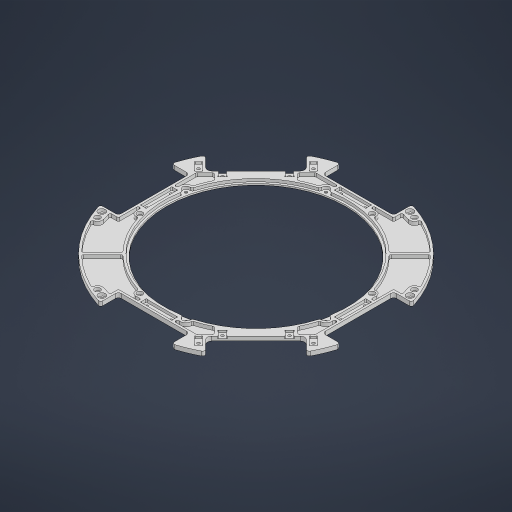
# Autodesk Inventor part: BasePlate
Saved by Autodesk Inventor 2024.2 (Build 282272000, 272)
## iProperties
Created: 2023-12-21
Part Number: BasePlate
Material: 一般
Document SubType Name: Modeling
Designer: Hanaoka
Density: 1 g/cm^3
Appearance: 既定
Author: Hanaoka
Autodesk Inventor part; units mm, degrees
(part 1 of 2)
ref_plane "YZ Plane" through (0, 0, 0) normal (1, 0, 0) x (0, 1, 0)
ref_plane "XZ Plane" through (0, 0, 0) normal (0, 1, 0) x (-1, 0, 0)
ref_plane "XY Plane" through (0, 0, 0) normal (0, 0, 1) x (1, 0, 0)
derived "MotorMount_main.ipt"
sketch "スケッチ4" plane through (-11, -15, 0) normal (0, -1, 0) x (1, 0, 0)
  circle A0 centre (19.5, 2) radius 0.8
  circle A1 centre (2.5, 2) radius 0.8
  line L0 (22, 0) -> (0, 0)
  line L1 (0, 0) -> (0, 4)
  line L2 (22, 4) -> (0, 4)
  line L3 (22, 0) -> (22, 4)
  circle A2 centre (11, -66) radius 90 construction
  line L4 (2.5, 2) -> (19.5, 2) construction
  line L5 (11, 2) -> (11, -66) construction
  circle A3 centre (11, -66) radius 88
  line L6 (-14, 18.374167) -> (-14, 7.5)
  line L7 (-12, 5.5) -> (34, 5.5)
  line L8 (36, 7.5) -> (36, 18.374167)
  arc A4 (-14, 7.5) -> (-12, 5.5) centre (-12, 7.5) ccw
  arc A5 (34, 5.5) -> (36, 7.5) centre (34, 7.5) ccw
  line L9 (0, 0) -> (22, 0)
  line L10 (22, 0) -> (22, 4)
  line L11 (22, 4) -> (0, 4)
  line L12 (0, 4) -> (0, 0)
  circle A6 centre (19.5, 2) radius 1
  circle A7 centre (2.5, 2) radius 1
  circle A8 centre (-57, -74.5) radius 1
  line L13 (-59, -77) -> (-55, -77)
  line L14 (-57, -74.5) -> (-57, -57.5) construction
  line L15 (-59, -55) -> (-59, -77)
  line L16 (-55, -55) -> (-59, -55)
  line L17 (-55, -77) -> (-55, -55)
  line L18 (-60.5, -89) -> (-60.5, -43)
  circle A9 centre (-57, -57.5) radius 1
  arc A10 (-62.5, -91) -> (-60.5, -89) centre (-62.5, -89) ccw
  line L19 (-62.5, -41) -> (-73.374167, -41)
  arc A11 (-60.5, -43) -> (-62.5, -41) centre (-62.5, -43) ccw
  line L20 (-73.374167, -91) -> (-62.5, -91)
  circle A12 centre (19.5, -134) radius 1
  line L21 (22, -136) -> (22, -132)
  line L22 (19.5, -134) -> (2.5, -134) construction
  line L23 (0, -136) -> (22, -136)
  line L24 (0, -132) -> (0, -136)
  line L25 (22, -132) -> (0, -132)
  line L26 (34, -137.5) -> (-12, -137.5)
  circle A13 centre (2.5, -134) radius 1
  arc A14 (36, -139.5) -> (34, -137.5) centre (34, -139.5) ccw
  line L27 (-14, -139.5) -> (-14, -150.374167)
  arc A15 (-12, -137.5) -> (-14, -139.5) centre (-12, -139.5) ccw
  line L28 (36, -150.374167) -> (36, -139.5)
  circle A16 centre (79, -57.5) radius 1
  line L29 (81, -55) -> (77, -55)
  line L30 (79, -57.5) -> (79, -74.5) construction
  line L31 (81, -77) -> (81, -55)
  line L32 (77, -77) -> (81, -77)
  line L33 (77, -55) -> (77, -77)
  line L34 (82.5, -43) -> (82.5, -89)
  circle A17 centre (79, -74.5) radius 1
  arc A18 (84.5, -41) -> (82.5, -43) centre (84.5, -43) ccw
  line L35 (84.5, -91) -> (95.374167, -91)
  arc A19 (82.5, -89) -> (84.5, -91) centre (84.5, -89) ccw
  line L36 (95.374167, -41) -> (84.5, -41)
  arc A20 (77.707107, -55) -> (77, -55.707107) centre (77.353553, -55.353553) ccw
  line L37 (77.353553, -55.353553) -> (77.353553, -55) construction
  line L38 (77.353553, -55.353553) -> (77, -55.353553) construction
  line L39 (77.353553, -55.353553) -> (77, -55) construction
  line L40 (80.646447, -55) -> (80.646447, -55.353553) construction
  line L41 (80.646447, -55.353553) -> (81, -55.353553) construction
  line L42 (77.353553, -77) -> (77.353553, -76.646447) construction
  line L43 (77.353553, -76.646447) -> (77, -76.646447) construction
  line L44 (81, -76.646447) -> (80.646447, -76.646447) construction
  line L45 (80.646447, -76.646447) -> (80.646447, -77) construction
  line L46 (81, -77) -> (80.646447, -76.646447) construction
  line L47 (77.353553, -76.646447) -> (77, -77) construction
  line L48 (81, -55) -> (80.646447, -55.353553) construction
  arc A21 (81, -55.707107) -> (80.292893, -55) centre (80.646447, -55.353553) ccw
  arc A22 (80.292893, -77) -> (81, -76.292893) centre (80.646447, -76.646447) ccw
  arc A23 (77, -76.292893) -> (77.707107, -77) centre (77.353553, -76.646447) ccw
  arc A24 (21.292893, 0) -> (22, 0.707107) centre (21.646447, 0.353553) ccw
  arc A25 (22, 3.292893) -> (21.292893, 4) centre (21.646447, 3.646447) ccw
  arc A26 (0, 0.707107) -> (0.707107, 0) centre (0.353553, 0.353553) ccw
  arc A27 (0.707107, 4) -> (0, 3.292893) centre (0.353553, 3.646447) ccw
  arc A28 (-55, -55.707107) -> (-55.707107, -55) centre (-55.353553, -55.353553) ccw
  arc A29 (-58.292893, -55) -> (-59, -55.707107) centre (-58.646447, -55.353553) ccw
  arc A30 (-55.707107, -77) -> (-55, -76.292893) centre (-55.353553, -76.646447) ccw
  arc A31 (-59, -76.292893) -> (-58.292893, -77) centre (-58.646447, -76.646447) ccw
  arc A32 (0.707107, -132) -> (0, -132.707107) centre (0.353553, -132.353553) ccw
  arc A33 (0, -135.292893) -> (0.707107, -136) centre (0.353553, -135.646447) ccw
  arc A34 (22, -132.707107) -> (21.292893, -132) centre (21.646447, -132.353553) ccw
  arc A35 (21.292893, -136) -> (22, -135.292893) centre (21.646447, -135.646447) ccw
  point P0 (11, 0)
  point P1 (-14, 5.5)
  point P2 (36, 5.5)
  point P3 (-57, -66)
  point P4 (-60.5, -91)
  point P5 (-60.5, -41)
  point P6 (11, -134)
  point P7 (36, -137.5)
  point P8 (-14, -137.5)
  point P9 (79, -66)
  point P10 (82.5, -41)
  point P11 (82.5, -91)
  point P12 (22, -135.292893)
  point P13 (21.292893, -136)
  point P14 (0.707107, -136)
  point P15 (0, -135.292893)
  point P16 (0, -132.707107)
  point P17 (0.707107, -132)
  point P18 (21.292893, -132)
  point P19 (22, -132.707107)
  point P20 (-58.292893, -77)
  point P21 (-59, -76.292893)
  point P22 (-59, -55.707107)
  point P23 (-58.292893, -55)
  point P24 (-55.707107, -55)
  point P25 (-55, -55.707107)
  point P26 (-55, -76.292893)
  point P27 (-55.707107, -77)
  point P28 (0, 3.292893)
  point P29 (0.707107, 4)
  point P30 (21.292893, 4)
  point P31 (22, 3.292893)
  point P32 (22, 0.707107)
  point P33 (21.292893, 0)
  point P34 (0.707107, 0)
  point P35 (0, 0.707107)
  dimension "d4" = 180
  dimension "d5" = 68
  dimension "d6" = 176
  dimension "d11" = 1.5
  dimension "d12" = 50
  dimension "d13" = 2
  dimension "d14" = 2
  dimension "d17" = 360
  dimension "d31" = 0.5
  dimension "d32" = 0.5
  dimension "d35" = 360
  constraints: 90 end point, 50 point on circle, 34 centre point, 32 point on line, 13 coincident, 8 equal length, 6 perpendicular, 5 equal radius, 4 horizontal, 4 tangent, 4 vertical, 3 parallel, 1 midpoint, 190 other
  measures "d4" diameter of A2
  measures "d5" distance of L5.start L5.end
  measures "d6" diameter of A3
  measures "d11" distance between parallel lines of L7 L2
  measures "d12" distance of point (-14, 5.5) point (36, 5.5)
  measures "d13" radius of A4
  measures "d14" diameter of A7
  measures "d31" radius of A20
  measures "d32" distance of L37.start L29.end
extrude "押し出し2" add sketch "スケッチ4" along normal blind 1 contours A24 L0 | L0 L1 L2 L3 | L3 A24 | A26 L0 | L3 A25 | A26 L1 | L2 A25 | A27 L1 | L2 A27 | L36 A18 L34 A19 L35 A3 L28 A14 L26 A15 L27 L20 A10 L18 A11 L19 L6 A4 L7 A5 L8 | A6 | A7 | L15 L16 L17 L13 | A31 L15 | L13 A31 | L13 A30 | A29 L15 | L17 A30 | A29 L16 | L17 A28 | A28 L16 | L23 L24 L25 L21 | A35 L23 | L21 A35 | L21 A34 | A33 L23 | L25 A34 | A33 L24 | L25 A32 | A32 L24 | L31 L32 L33 L29 | A21 L31 | L29 A21 | L29 A20 | A22 L31 | L33 A20 | A22 L32 | L33 A23 | A23 L32
extrude "押し出し3" add sketch "スケッチ4" against normal blind 2 contours L36 A18 L34 A19 L35 A3 L28 A14 L26 A15 L27 L20 A10 L18 A11 L19 L6 A4 L7 A5 L8
fillet "フィレット1" radius 1.5 8 edges at (-84.3742, -14.5, -41) (-25, -14.5, 18.3742) (25, -14.5, 18.3742) (84.3742, -14.5, -41) (84.3742, -14.5, -91) (25, -14.5, -150.3742) (-25, -14.5, -150.3742) (-84.3742, -14.5, -91)
sketch "溝切り" plane through (-23, -13, 5.5) normal (0, 1, 0) x (1, 0, 0)
  circle A0 centre (102.548727, 100) radius 2.5
  line L0 (96.5, 96.5) -> (105.340755, 96.5)
  arc A1 (106.76863, 98.459538) -> (49.959538, 155.26863) centre (23, 71.5) ccw
  circle A2 centre (102.548727, 100) radius 3.5 construction
  line L1 (85.225397, 133.725397) -> (-39.225397, 9.274603) construction
  arc A3 (-60.76863, 44.540462) -> (-3.959538, -12.26863) centre (23, 71.5) ccw
  circle A4 centre (51.5, 151.048727) radius 2.5
  circle A5 centre (51.5, 151.048727) radius 3.5 construction
  line L2 (-39.225397, 133.725397) -> (85.225397, 9.274603) construction
  arc A6 (49.959538, -12.26863) -> (106.76863, 44.540462) centre (23, 71.5) ccw
  arc A7 (-3.959538, 155.26863) -> (-60.76863, 98.459538) centre (23, 71.5) ccw
  circle A8 centre (-5.5, -8.048727) radius 2.5
  circle A9 centre (-5.5, -8.048727) radius 3.5 construction
  circle A10 centre (-56.548727, 43) radius 3.5 construction
  circle A11 centre (-56.548727, 43) radius 2.5
  circle A12 centre (102.548727, 100) radius 1.3
  circle A13 centre (51.5, 151.048727) radius 1.3
  circle A14 centre (-56.548727, 43) radius 1.3
  circle A15 centre (-5.5, -8.048727) radius 1.3
  circle A16 centre (23, 71.5) radius 63
  line L3 (-54.339215, 113.483876) -> (-46.914594, 106.059255)
  line L4 (-42.671953, 106.059255) -> (-11.559255, 137.171953)
  line L5 (-11.559255, 141.414594) -> (-18.983876, 148.839215)
  arc A17 (-46.914594, 106.059255) -> (-42.671953, 106.059255) centre (-44.793273, 108.180575) ccw
  arc A18 (-11.559255, 137.171953) -> (-11.559255, 141.414594) centre (-13.680575, 139.293273) ccw
  circle A19 centre (-41.964846, 136.464846) radius 21 construction
  line L6 (64.983876, -5.839215) -> (57.559255, 1.585406)
  line L7 (57.559255, 5.828047) -> (88.671953, 36.940745)
  line L8 (92.914594, 36.940745) -> (100.339215, 29.516124)
  arc A20 (57.559255, 5.828047) -> (57.559255, 1.585406) centre (59.680575, 3.706727) ccw
  arc A21 (92.914594, 36.940745) -> (88.671953, 36.940745) centre (90.793273, 34.819425) ccw
  circle A22 centre (8.265706, 135.321239) radius 2.5 construction
  circle A23 centre (8.265706, 135.321239) radius 1
  line L9 (8.265706, 135.321239) -> (23, 71.5) construction
  arc A24 (10.701631, 135.883617) -> (5.829781, 134.758862) centre (8.265706, 135.321239) ccw
  line L10 (5.829781, 134.758862) -> (6.403321, 132.274586)
  line L11 (10.701631, 135.883617) -> (11.275171, 133.399341)
  circle A25 centre (-40.821239, 86.234294) radius 2.5 construction
  circle A26 centre (-40.821239, 86.234294) radius 1
  arc A27 (-40.258862, 88.670219) -> (-41.383617, 83.798369) centre (-40.821239, 86.234294) ccw
  line L12 (-40.258862, 88.670219) -> (-37.774586, 88.096679)
  line L13 (-41.383617, 83.798369) -> (-38.899341, 83.224829)
  circle A28 centre (86.821239, 56.765706) radius 2.5 construction
  circle A29 centre (86.821239, 56.765706) radius 1
  arc A30 (86.258862, 54.329781) -> (87.383617, 59.201631) centre (86.821239, 56.765706) ccw
  line L14 (86.258862, 54.329781) -> (83.774586, 54.903321)
  line L15 (87.383617, 59.201631) -> (84.899341, 59.775171)
  line L16 (35.298369, 7.116383) -> (34.724829, 9.600659)
  line L17 (40.170219, 8.241138) -> (39.596679, 10.725414)
  circle A31 centre (37.734294, 7.678761) radius 2.5 construction
  circle A32 centre (37.734294, 7.678761) radius 1
  arc A33 (35.298369, 7.116383) -> (40.170219, 8.241138) centre (37.734294, 7.678761) ccw
  circle A34 centre (23, 71.5) radius 64.5
  line L18 (-48.5, 94.5) -> (-48.5, 96.330952) construction
  line L19 (-48.5, 96.330952) -> (-58.01901, 105.849963) construction
  line L20 (-48.5, 94.5) -> (-48.5, 48.5)
  line L21 (0, 143) -> (-1.830952, 143) construction
  line L22 (-1.830952, 143) -> (-11.349963, 152.51901) construction
  arc A35 (-60.76863, 98.459538) -> (-59.340755, 96.5) centre (-59.340755, 98) ccw
  line L23 (-59.340755, 96.5) -> (-50.5, 96.5)
  arc A36 (-48.5, 94.5) -> (-50.5, 96.5) centre (-50.5, 94.5) ccw
  arc A37 (-2, 153.840755) -> (-3.959538, 155.26863) centre (-3.5, 153.840755) ccw
  line L24 (-2, 145) -> (-2, 153.840755)
  arc A38 (-2, 145) -> (0, 143) centre (0, 145) ccw
  line L25 (46, 143) -> (0, 143)
  point P0 (23, 5.5)
  point P1 (-44.793273, 103.937934)
  point P2 (-9.437934, 139.293273)
  point P3 (100.339215, 29.516124)
  point P4 (39.596679, 10.725414)
  point P5 (34.724829, 9.600659)
  point P6 (84.899341, 59.775171)
  point P7 (83.774586, 54.903321)
  point P8 (-38.899341, 83.224829)
  point P9 (-37.774586, 88.096679)
  point P10 (-40.362021, 83.562515)
  point P11 (35.062515, 8.137979)
  point P12 (39.934365, 9.262734)
  point P13 (85.237266, 54.565635)
  point P14 (86.362021, 59.437485)
  point P15 (10.937485, 134.862021)
  point P16 (6.065635, 133.737266)
  point P17 (-39.237266, 88.434365)
  point P18 (-50.626904, 109.771565)
  point P19 (-11.349963, 152.51901)
  dimension "d20" = 5
  dimension "d22" = 7
  dimension "d23" = 2.6
  dimension "d28" = 126
  dimension "d37" = 50
  dimension "d38" = 3
  dimension "d39" = 42
  dimension "d40" = 13.5
  dimension "d45" = 2
  dimension "d46" = 5
  dimension "d47" = 32
  dimension "d48" = 1.5
  dimension "d102" = 8
  constraints: 42 end point, 38 symmetric about line, 31 centre point, 25 point on circle, 18 coincident, 11 tangent, 7 parallel, 5 equal radius, 5 point on line, 2 midpoint, 1 collinear, 1 vertical, 17 other
  measures "d20" diameter of A0
  measures "d22" diameter of A2
  measures "d23" diameter of A12
  measures "d28" diameter of A16
  measures "d37" distance of point (-44.793, 103.938) point (-9.438, 139.293)
  measures "d38" radius of A17
  measures "d39" diameter of A19
  measures "d40" distance from line of L5.end L4
  measures "d45" diameter of A23
  measures "d46" diameter of A22
  measures "d47" angle of L2 L9
  measures "d48" radial gap between concentric circles of A16 A34
  measures "d102" distance from line of point (-50.627, 109.772) L19
extrude "押し出し4" cut sketch "溝切り" against normal up to surface (3 mm away) contours A12 | A13 | A14 | A15
extrude "押し出し5" cut sketch "溝切り" against normal blind 2 contours A0 | A4 | A8 | A11 | A15 | A16 | A16 L11 A34 L15 | A16 L10 A34 L11 | L15 A34 L14 A16 | A16 L12 A34 L10 | A34 L10 A24 L11 | L14 A34 L17 A16 | L15 A30 L14 A34 | A16 L13 A34 L12 | L17 A34 L16 A16 | A16 L16 A34 L13 | A34 L13 A27 L12 | L17 A33 L16 A34
extrude "押し出し6" cut sketch "溝切り" against normal up to surface (3 mm away) contours L6 A20 L7 A21 L8 A6 | L5 A18 L4 A17 L3 A7 | A16 | A23 | A29 | A32 | A26
fillet "フィレット2" radius 1.5 4 edges at (-77.3392, -14.5, -107.9839) (-41.9839, -14.5, -143.3392) (41.9839, -14.5, 11.3392) (77.3392, -14.5, -24.0161)
fillet "フィレット3" radius 1.5 8 edges at (-62.2373, -14, -82.9344) (-63.362, -14, -78.0625) (-16.9344, -14, -128.2373) (-12.0625, -14, -129.362) (63.362, -14, -53.9375) (62.2373, -14, -49.0656) (12.0625, -14, -2.638) (16.9344, -14, -3.7627)
sketch "シャフト用はめ穴" plane through (-23, -13, -137.5) normal (0, 1, 0) x (1, 0, 0)
  circle A0 centre (-54.526174, -105.114614) radius 1
  circle A1 centre (-54.526174, -105.114614) radius 2
  circle A2 centre (-41.936507, -88) radius 2
  circle A3 centre (-41.936507, -88) radius 1
  circle A4 centre (-56.548727, -100) radius 2.5
  circle A5 centre (23, -71.5) radius 63
  arc A6 (-56.548727, -100) -> (-54.526174, -105.114614) centre (23, -71.5) ccw construction
  line L0 (85.225397, -9.274603) -> (-39.225397, -133.725397) construction
  line L1 (-39.225397, -9.274603) -> (85.225397, -133.725397) construction
  circle A7 centre (-10.614614, -149.026174) radius 1
  circle A8 centre (-10.614614, -149.026174) radius 2
  circle A9 centre (-41.936507, -88) radius 2.5 construction
  arc A10 (-40.607766, -60.808783) -> (33.691217, -135.107766) centre (23, -71.5) ccw
  line L2 (-43.707107, -82.5) -> (-46.292893, -82.5)
  circle A11 centre (6.5, -136.436507) radius 2
  circle A12 centre (6.5, -136.436507) radius 1
  circle A13 centre (6.5, -136.436507) radius 2.5 construction
  circle A14 centre (56.614614, 6.026174) radius 1
  circle A15 centre (56.614614, 6.026174) radius 2
  circle A16 centre (39.5, -6.563493) radius 2
  circle A17 centre (39.5, -6.563493) radius 1
  circle A18 centre (100.526174, -37.885386) radius 1
  circle A19 centre (100.526174, -37.885386) radius 2
  circle A20 centre (87.936507, -55) radius 2
  circle A21 centre (87.936507, -55) radius 1
  point P0 (23, -137.5)
  dimension "d50" = 2
  dimension "d51" = 4
  dimension "d52" = 1
  dimension "d53" = 5
  dimension "d54" = 3
  constraints: 19 centre point, 13 symmetric about line, 12 coincident, 2 equal radius, 2 point on circle, 1 tangent, 13 other
  measures "d50" diameter of A0
  measures "d51" diameter of A1
  measures "d53" diameter of A9
  measures "d54" distance edge to line of A9 L2
extrude "押し出し7" cut sketch "シャフト用はめ穴" against normal up to surface (2 mm away) contours A0 | A1 | A2 | A3 | A7 | A8 | A11 | A12 | A14 | A15 | A16 | A17 | A18 | A19 | A20 | A21
extrude "押し出し8" cut sketch "シャフト用はめ穴" against normal up to surface (3 mm away) contours A0 | A3 | A7 | A12 | A14 | A17 | A18 | A21
sketch "キッカー用はめあい" plane through (-23, -13, -137.5) normal (0, 1, 0) x (1, 0, 0)
  circle A0 centre (83.121165, -108.074509) radius 1
  circle A1 centre (59.574509, -131.621165) radius 1
  line L0 (88.671953, -106.059255) -> (57.559255, -137.171953)
  line L1 (73.115604, -121.615604) -> (68.608387, -117.108387) construction
  line L2 (57.559255, -137.171953) -> (88.671953, -106.059255)
  arc A2 (41.274607, -133.357002) -> (84.857002, -89.774607) centre (23, -71.5) ccw
  line L3 (59.574509, -131.621165) -> (83.121165, -108.074509) construction
  line L4 (86.303145, -108.428062) -> (82.767611, -104.892528)
  line L5 (82.767611, -104.892528) -> (79.939184, -107.720956)
  line L6 (79.939184, -107.720956) -> (83.474718, -111.25649)
  circle A3 centre (83.121165, -108.074509) radius 2 construction
  line L7 (59.928062, -134.803145) -> (56.392528, -131.267611)
  line L8 (56.392528, -131.267611) -> (59.220956, -128.439184)
  line L9 (59.220956, -128.439184) -> (62.75649, -131.974718)
  arc A4 (83.474718, -105.599635) -> (82.767611, -104.892528) centre (83.121165, -105.246082) ccw
  line L10 (82.767611, -104.892528) -> (83.121165, -105.246082)
  line L11 (79.939184, -107.720956) -> (80.292738, -108.074509)
  arc A5 (79.939184, -107.720956) -> (80.646291, -108.428062) centre (80.292738, -108.074509) ccw
  arc A6 (56.392528, -131.267611) -> (57.099635, -131.974718) centre (56.746082, -131.621165) ccw
  arc A7 (59.928062, -129.146291) -> (59.220956, -128.439184) centre (59.574509, -128.792738) ccw
  line L12 (-21.547727, -116.047727) -> (67.547727, -26.952273) construction
  circle A8 centre (23, -71.5) radius 63
  circle A9 centre (-13.574509, -11.378835) radius 1
  circle A10 centre (-37.121165, -34.925491) radius 1
  line L13 (-27.115604, -21.384396) -> (-22.608387, -25.891613) construction
  line L14 (-37.121165, -34.925491) -> (-13.574509, -11.378835) construction
  line L15 (-13.928062, -8.196855) -> (-10.392528, -11.732389)
  line L16 (-10.392528, -11.732389) -> (-13.220956, -14.560816)
  line L17 (-13.220956, -14.560816) -> (-16.75649, -11.025282)
  circle A11 centre (-13.574509, -11.378835) radius 2 construction
  line L18 (-40.303145, -34.571938) -> (-36.767611, -38.107472)
  line L19 (-36.767611, -38.107472) -> (-33.939184, -35.279044)
  line L20 (-33.939184, -35.279044) -> (-37.474718, -31.74351)
  arc A12 (-10.392528, -11.732389) -> (-11.099635, -11.025282) centre (-10.746082, -11.378835) ccw
  line L21 (-10.392528, -11.732389) -> (-10.746082, -11.378835)
  line L22 (-13.220956, -14.560816) -> (-13.574509, -14.207262)
  arc A13 (-13.928062, -13.853709) -> (-13.220956, -14.560816) centre (-13.574509, -14.207262) ccw
  arc A14 (-37.474718, -37.400365) -> (-36.767611, -38.107472) centre (-37.121165, -37.753918) ccw
  arc A15 (-33.939184, -35.279044) -> (-34.646291, -34.571938) centre (-34.292738, -34.925491) ccw
  line L23 (-40.303145, -34.571938) -> (-37.474718, -31.74351)
  line L24 (-42.671953, -36.940745) -> (-11.559255, -5.828047)
  line L25 (-16.75649, -11.025282) -> (-13.928062, -8.196855)
  line L26 (-54.339215, -37.294299) -> (-51.510788, -34.465872)
  line L27 (-51.510788, -34.465872) -> (-45.853934, -40.122726)
  line L28 (-45.853934, -40.122726) -> (-48.682361, -42.951153)
  line L29 (-48.682361, -42.951153) -> (-54.339215, -37.294299)
  line L30 (-46.914594, -36.940745) -> (-52.901376, -30.953963)
  line L31 (-11.559255, -5.828047) -> (-42.671953, -36.940745)
  circle A16 centre (-50.096574, -38.708512) radius 1
  line L32 (-51.510788, -40.122726) -> (-48.682361, -37.294299) construction
  line L33 (-47.268147, -41.536939) -> (-52.925001, -35.880085) construction
  arc A17 (-53.839215, -36.794299) -> (-53.839215, -37.794299) centre (-53.839215, -37.294299) ccw
  line L34 (-54.339215, -37.294299) -> (-53.839215, -37.294299) construction
  line L35 (-53.839215, -37.294299) -> (-54.089215, -37.044299) construction
  line L36 (-53.839215, -37.294299) -> (-54.089215, -37.544299) construction
  arc A18 (-51.010788, -34.965872) -> (-52.010788, -34.965872) centre (-51.510788, -34.965872) ccw
  arc A19 (-49.182361, -42.451153) -> (-48.182361, -42.451153) centre (-48.682361, -42.451153) ccw
  arc A20 (-46.353934, -40.622726) -> (-46.353934, -39.622726) centre (-46.353934, -40.122726) ccw
  line L37 (-11.205701, 5.839215) -> (-14.034128, 3.010788)
  line L38 (-14.034128, 3.010788) -> (-8.377274, -2.646066)
  line L39 (-8.377274, -2.646066) -> (-5.548847, 0.182361)
  line L40 (-5.548847, 0.182361) -> (-11.205701, 5.839215)
  circle A21 centre (-9.791488, 1.596574) radius 1
  arc A22 (-10.705701, 5.339215) -> (-11.705701, 5.339215) centre (-11.205701, 5.339215) ccw
  arc A23 (-13.534128, 3.510788) -> (-13.534128, 2.510788) centre (-13.534128, 3.010788) ccw
  arc A24 (-6.048847, -0.317639) -> (-6.048847, 0.682361) centre (-6.048847, 0.182361) ccw
  arc A25 (-8.877274, -2.146066) -> (-7.877274, -2.146066) centre (-8.377274, -2.146066) ccw
  line L41 (57.205701, -148.839215) -> (60.034128, -146.010788)
  line L42 (60.034128, -146.010788) -> (54.377274, -140.353934)
  line L43 (54.377274, -140.353934) -> (51.548847, -143.182361)
  line L44 (51.548847, -143.182361) -> (57.205701, -148.839215)
  circle A26 centre (55.791488, -144.596574) radius 1
  arc A27 (56.705701, -148.339215) -> (57.705701, -148.339215) centre (57.205701, -148.339215) ccw
  arc A28 (59.534128, -146.510788) -> (59.534128, -145.510788) centre (59.534128, -146.010788) ccw
  arc A29 (52.048847, -142.682361) -> (52.048847, -143.682361) centre (52.048847, -143.182361) ccw
  arc A30 (54.877274, -140.853934) -> (53.877274, -140.853934) centre (54.377274, -140.853934) ccw
  line L45 (94.682361, -100.048847) -> (100.339215, -105.705701)
  arc A31 (99.839215, -106.205701) -> (99.839215, -105.205701) centre (99.839215, -105.705701) ccw
  line L46 (100.339215, -105.705701) -> (97.510788, -108.534128)
  arc A32 (97.010788, -108.034128) -> (98.010788, -108.034128) centre (97.510788, -108.034128) ccw
  line L47 (97.510788, -108.534128) -> (91.853934, -102.877274)
  circle A33 centre (96.096574, -104.291488) radius 1
  line L48 (91.853934, -102.877274) -> (94.682361, -100.048847)
  arc A34 (95.182361, -100.548847) -> (94.182361, -100.548847) centre (94.682361, -100.548847) ccw
  arc A35 (92.353934, -102.377274) -> (92.353934, -103.377274) centre (92.353934, -102.877274) ccw
  point P0 (23, -137.5)
  point P1 (86.303145, -108.428062)
  point P2 (59.928062, -129.146291)
  point P3 (59.220956, -128.439184)
  point P4 (57.099635, -131.974718)
  point P5 (-13.220956, -14.560816)
  point P6 (-10.392528, -11.732389)
  point P7 (-36.767611, -38.107472)
  point P8 (-34.646291, -34.571938)
  point P9 (-37.474718, -37.400365)
  point P10 (95.182361, -100.548847)
  point P11 (94.182361, -100.548847)
  point P12 (92.353934, -102.377274)
  point P13 (92.353934, -103.377274)
  point P14 (97.010788, -108.034128)
  point P15 (98.010788, -108.034128)
  point P16 (53.877274, -140.853934)
  point P17 (52.048847, -142.682361)
  point P18 (52.048847, -143.682361)
  point P19 (59.534128, -146.510788)
  point P20 (59.534128, -145.510788)
  point P21 (54.877274, -140.853934)
  point P22 (-7.877274, -2.146066)
  point P23 (-6.048847, -0.317639)
  point P24 (-6.048847, 0.682361)
  point P25 (-13.534128, 3.510788)
  point P26 (-13.534128, 2.510788)
  point P27 (-8.877274, -2.146066)
  point P28 (-48.182361, -42.451153)
  point P29 (-46.353934, -40.622726)
  point P30 (-46.353934, -39.622726)
  point P31 (-51.010788, -34.965872)
  point P32 (-52.010788, -34.965872)
  point P33 (-49.182361, -42.451153)
  dimension "d59" = 2
  dimension "d60" = 33.3
  dimension "d61" = 2.5
  dimension "d62" = 4
  dimension "d63" = 5
  dimension "d68" = 0.5
  dimension "d69" = 0.5
  dimension "d84" = 8
  dimension "d85" = 4
  dimension "d86" = 1.5
  dimension "d88" = 2
  dimension "d89" = 0.5
  dimension "d90" = 0.5
  constraints: 100 symmetric about line, 88 end point, 51 point on circle, 34 centre point, 33 point on line, 8 coincident, 7 midpoint, 7 parallel, 7 perpendicular, 2 collinear, 2 equal radius, 2 tangent, 1 horizontal, 28 other
  measures "d59" diameter of A0
  measures "d60" distance of L3.start L3.end
  measures "d61" distance between parallel lines of L0 L3
  measures "d62" diameter of A3
  measures "d63" distance of L4.start L4.end
  measures "d68" distance of L4.end L10.end
  measures "d69" radius of A4
  measures "d84" distance of L28.end L29.end
  measures "d85" distance of L26.start L26.end
  measures "d86" distance between parallel lines of L30 L27
  measures "d88" diameter of A16
  measures "d89" distance of L26.start L34.end
  measures "d90" radius of A17
extrude "押し出し9" cut sketch "キッカー用はめあい" against normal blind 1.5 contours A0 | A1 | L0 L6 L5 L4 | L4 A4 | A5 L6 | L0 L7 L8 L9 | L9 A7 | A6 L7 | A9 | A10 | L15 L16 L17 L24 | A12 L15 | L17 A13 | L23 L20 L19 L18 | L18 A14 | A15 L20 | A17 L26 | L26 L27 L28 L29 | L29 A17 | A18 L26 | L29 A19 | A18 L27 | L28 A19 | A20 L27 | L28 A20 | A16 | L40 L39 L38 L37 | A22 L40 | L37 A22 | L37 A23 | A24 L40 | L38 A23 | A24 L39 | L38 A25 | A25 L39 | A21 | L44 L43 L42 L41 | A27 L44 | L41 A27 | L41 A28 | A29 L44 | L42 A28 | A29 L43 | L42 A30 | A30 L43 | A26 | A34 L45 | L45 L46 L47 L48 | L48 A34 | A31 L45 | L48 A35 | A31 L46 | L47 A35 | A32 L46 | L47 A32 | A33
extrude "押し出し10" cut sketch "キッカー用はめあい" against normal up to surface (3 mm away) contours A0 | A1 | A9 | A10 | A16 | A21 | A26 | A33
fillet "フィレット4" radius 0.5 8 edges at (36.9281, -13.75, -2.6969) (39.7565, -13.75, -5.5253) (60.4747, -13.75, -26.2435) (63.3031, -13.75, -29.0719) (-63.3031, -13.75, -102.9281) (-60.4747, -13.75, -105.7565) (-39.7565, -13.75, -126.4747) (-36.9281, -13.75, -129.3031)
sketch "肉抜き" plane through (-23, -13, 5.5) normal (0, 1, 0) x (1, 0, 0)
  circle A0 centre (102.548727, 100) radius 2.5
  circle A1 centre (-5.5, -8.048727) radius 2.5
  circle A2 centre (51.5, 151.048727) radius 2.5
  circle A3 centre (-56.548727, 43) radius 2.5
  arc A4 (41.274607, 9.642998) -> (40.212609, 8.007325) centre (41.699598, 8.204463) ccw
  arc A5 (35.362766, 6.88765) -> (40.212609, 8.007325) centre (37.734294, 7.678761) ccw
  arc A6 (35.362766, 6.88765) -> (33.691217, 7.892234) centre (33.93985, 6.412984) ccw
  arc A7 (-40.607766, 82.191217) -> (33.691217, 7.892234) centre (23, 71.5) ccw
  arc A8 (-40.607766, 82.191217) -> (-41.61235, 83.862766) centre (-42.087016, 82.43985) ccw
  arc A9 (-40.492675, 88.712609) -> (-41.61235, 83.862766) centre (-40.821239, 86.234294) ccw
  arc A10 (-40.492675, 88.712609) -> (-38.857002, 89.774607) centre (-40.295537, 90.199598) ccw
  arc A11 (4.725393, 133.357002) -> (-38.857002, 89.774607) centre (23, 71.5) ccw
  arc A12 (4.725393, 133.357002) -> (5.787391, 134.992675) centre (4.300402, 134.795537) ccw
  arc A13 (10.637234, 136.11235) -> (5.787391, 134.992675) centre (8.265706, 135.321239) ccw
  arc A14 (10.637234, 136.11235) -> (12.308783, 135.107766) centre (12.06015, 136.587016) ccw
  arc A15 (86.607766, 60.808783) -> (12.308783, 135.107766) centre (23, 71.5) ccw
  arc A16 (86.607766, 60.808783) -> (87.61235, 59.137234) centre (88.087016, 60.56015) ccw
  arc A17 (86.492675, 54.287391) -> (87.61235, 59.137234) centre (86.821239, 56.765706) ccw
  arc A18 (86.492675, 54.287391) -> (84.857002, 53.225393) centre (86.295537, 52.800402) ccw
  arc A19 (41.274607, 9.642998) -> (84.857002, 53.225393) centre (23, 71.5) ccw
  arc A20 (34, 140.792893) -> (33.292893, 141.5) centre (33.646447, 141.146447) ccw
  line L0 (34, 140.792893) -> (34, 138.207107)
  arc A21 (33.292893, 137.5) -> (34, 138.207107) centre (33.646447, 137.853553) ccw
  line L1 (33.292893, 137.5) -> (12.707107, 137.5)
  arc A22 (12, 138.207107) -> (12.707107, 137.5) centre (12.353553, 137.853553) ccw
  line L2 (12, 138.207107) -> (12, 140.792893)
  arc A23 (12.707107, 141.5) -> (12, 140.792893) centre (12.353553, 141.146447) ccw
  line L3 (12.707107, 141.5) -> (33.292893, 141.5)
  arc A24 (-46.292893, 82.5) -> (-47, 81.792893) centre (-46.646447, 82.146447) ccw
  line L4 (-46.292893, 82.5) -> (-43.707107, 82.5)
  arc A25 (-43, 81.792893) -> (-43.707107, 82.5) centre (-43.353553, 82.146447) ccw
  line L5 (-43, 81.792893) -> (-43, 61.207107)
  arc A26 (-43.707107, 60.5) -> (-43, 61.207107) centre (-43.353553, 60.853553) ccw
  line L6 (-43.707107, 60.5) -> (-46.292893, 60.5)
  arc A27 (-47, 61.207107) -> (-46.292893, 60.5) centre (-46.646447, 60.853553) ccw
  line L7 (-47, 61.207107) -> (-47, 81.792893)
  arc A28 (12, 2.207107) -> (12.707107, 1.5) centre (12.353553, 1.853553) ccw
  line L8 (12, 2.207107) -> (12, 4.792893)
  arc A29 (12.707107, 5.5) -> (12, 4.792893) centre (12.353553, 5.146447) ccw
  line L9 (12.707107, 5.5) -> (33.292893, 5.5)
  arc A30 (34, 4.792893) -> (33.292893, 5.5) centre (33.646447, 5.146447) ccw
  line L10 (34, 4.792893) -> (34, 2.207107)
  arc A31 (33.292893, 1.5) -> (34, 2.207107) centre (33.646447, 1.853553) ccw
  line L11 (33.292893, 1.5) -> (12.707107, 1.5)
  arc A32 (89.707107, 82.5) -> (89, 81.792893) centre (89.353553, 82.146447) ccw
  line L12 (89.707107, 82.5) -> (92.292893, 82.5)
  arc A33 (93, 81.792893) -> (92.292893, 82.5) centre (92.646447, 82.146447) ccw
  line L13 (93, 81.792893) -> (93, 61.207107)
  arc A34 (92.292893, 60.5) -> (93, 61.207107) centre (92.646447, 60.853553) ccw
  line L14 (92.292893, 60.5) -> (89.707107, 60.5)
  arc A35 (89, 61.207107) -> (89.707107, 60.5) centre (89.353553, 60.853553) ccw
  line L15 (89, 61.207107) -> (89, 81.792893)
  circle A36 centre (-41.936507, 55) radius 2
  circle A37 centre (6.5, 6.563493) radius 2
  circle A38 centre (-54.526174, 37.885386) radius 2
  circle A39 centre (-10.614614, -6.026174) radius 2
  arc A40 (-13.574509, 135.156699) -> (-13.574509, 134.449592) centre (-13.220956, 134.803145) ccw
  line L16 (-13.574509, 134.449592) -> (-11.099635, 131.974718)
  arc A41 (-10.392528, 131.267611) -> (-11.099635, 131.974718) centre (-10.746082, 131.621165) ccw
  line L17 (-10.392528, 131.267611) -> (-13.220956, 128.439184)
  arc A42 (-13.928062, 129.146291) -> (-13.220956, 128.439184) centre (-13.574509, 128.792738) ccw
  line L18 (-13.928062, 129.146291) -> (-16.402936, 131.621165)
  arc A43 (-16.402936, 131.621165) -> (-17.110043, 131.621165) centre (-16.75649, 131.267611) ccw
  line L19 (-17.110043, 131.621165) -> (-37.121165, 111.610043)
  arc A44 (-37.121165, 111.610043) -> (-37.121165, 110.902936) centre (-36.767611, 111.25649) ccw
  line L20 (-37.121165, 110.902936) -> (-34.646291, 108.428062)
  arc A45 (-33.939184, 107.720956) -> (-34.646291, 108.428062) centre (-34.292738, 108.074509) ccw
  line L21 (-33.939184, 107.720956) -> (-36.767611, 104.892528)
  arc A46 (-37.474718, 105.599635) -> (-36.767611, 104.892528) centre (-37.121165, 105.246082) ccw
  line L22 (-37.474718, 105.599635) -> (-39.949592, 108.074509)
  arc A47 (-39.949592, 108.074509) -> (-40.656699, 108.074509) centre (-40.303145, 107.720956) ccw
  line L23 (-40.656699, 108.074509) -> (-42.671953, 106.059255)
  arc A48 (-46.914594, 106.059255) -> (-42.671953, 106.059255) centre (-44.793273, 108.180575) ccw
  line L24 (-46.914594, 106.059255) -> (-52.901376, 112.046037)
  arc A49 (-52.901376, 112.046037) -> (-55.296638, 111.670094) centre (-53.962036, 110.985377) ccw
  arc A50 (-55.296638, 111.670094) -> (-60.76863, 98.459538) centre (23, 71.5) ccw
  line L25 (-48.5, 94.5) -> (-48.5, 48.5)
  arc A51 (-50.5, 46.5) -> (-48.5, 48.5) centre (-50.5, 48.5) ccw
  line L26 (-50.5, 46.5) -> (-59.340755, 46.5)
  arc A52 (-59.340755, 46.5) -> (-60.76863, 44.540462) centre (-59.340755, 45) ccw
  arc A53 (-60.76863, 44.540462) -> (-3.959538, -12.26863) centre (23, 71.5) ccw
  arc A54 (-3.959538, -12.26863) -> (-2, -10.840755) centre (-3.5, -10.840755) ccw
  line L27 (-2, -10.840755) -> (-2, -2)
  arc A55 (0, 0) -> (-2, -2) centre (0, -2) ccw
  line L28 (0, 0) -> (46, 0)
  arc A56 (48, -2) -> (46, 0) centre (46, -2) ccw
  line L29 (48, -2) -> (48, -10.840755)
  arc A57 (48, -10.840755) -> (49.959538, -12.26863) centre (49.5, -10.840755) ccw
  arc A58 (49.959538, -12.26863) -> (63.170094, -6.796638) centre (23, 71.5) ccw
  arc A59 (63.170094, -6.796638) -> (63.546037, -4.401376) centre (62.485377, -5.462036) ccw
  line L30 (63.546037, -4.401376) -> (57.559255, 1.585406)
  arc A60 (57.559255, 5.828047) -> (57.559255, 1.585406) centre (59.680575, 3.706727) ccw
  line L31 (57.559255, 5.828047) -> (59.574509, 7.843301)
  arc A61 (59.574509, 7.843301) -> (59.574509, 8.550408) centre (59.220956, 8.196855) ccw
  line L32 (59.574509, 8.550408) -> (57.099635, 11.025282)
  arc A62 (56.392528, 11.732389) -> (57.099635, 11.025282) centre (56.746082, 11.378835) ccw
  line L33 (56.392528, 11.732389) -> (59.220956, 14.560816)
  arc A63 (59.928062, 13.853709) -> (59.220956, 14.560816) centre (59.574509, 14.207262) ccw
  line L34 (59.928062, 13.853709) -> (62.402936, 11.378835)
  arc A64 (62.402936, 11.378835) -> (63.110043, 11.378835) centre (62.75649, 11.732389) ccw
  line L35 (63.110043, 11.378835) -> (83.121165, 31.389957)
  arc A65 (83.121165, 31.389957) -> (83.121165, 32.097064) centre (82.767611, 31.74351) ccw
  line L36 (83.121165, 32.097064) -> (80.646291, 34.571938)
  arc A66 (79.939184, 35.279044) -> (80.646291, 34.571938) centre (80.292738, 34.925491) ccw
  line L37 (79.939184, 35.279044) -> (82.767611, 38.107472)
  arc A67 (83.474718, 37.400365) -> (82.767611, 38.107472) centre (83.121165, 37.753918) ccw
  line L38 (83.474718, 37.400365) -> (85.949592, 34.925491)
  arc A68 (85.949592, 34.925491) -> (86.656699, 34.925491) centre (86.303145, 35.279044) ccw
  line L39 (86.656699, 34.925491) -> (88.671953, 36.940745)
  arc A69 (92.914594, 36.940745) -> (88.671953, 36.940745) centre (90.793273, 34.819425) ccw
  line L40 (92.914594, 36.940745) -> (98.901376, 30.953963)
  arc A70 (98.901376, 30.953963) -> (101.296638, 31.329906) centre (99.962036, 32.014623) ccw
  arc A71 (101.296638, 31.329906) -> (106.76863, 44.540462) centre (23, 71.5) ccw
  arc A72 (106.76863, 44.540462) -> (105.340755, 46.5) centre (105.340755, 45) ccw
  line L41 (105.340755, 46.5) -> (96.5, 46.5)
  arc A73 (94.5, 48.5) -> (96.5, 46.5) centre (96.5, 48.5) ccw
  line L42 (94.5, 48.5) -> (94.5, 94.5)
  arc A74 (96.5, 96.5) -> (94.5, 94.5) centre (96.5, 94.5) ccw
  line L43 (96.5, 96.5) -> (105.340755, 96.5)
  arc A75 (105.340755, 96.5) -> (106.76863, 98.459538) centre (105.340755, 98) ccw
  arc A76 (106.76863, 98.459538) -> (49.959538, 155.26863) centre (23, 71.5) ccw
  arc A77 (49.959538, 155.26863) -> (48, 153.840755) centre (49.5, 153.840755) ccw
  line L44 (48, 153.840755) -> (48, 145)
  arc A78 (46, 143) -> (48, 145) centre (46, 145) ccw
  line L45 (46, 143) -> (0, 143)
  arc A79 (-3.959538, 155.26863) -> (-17.170094, 149.796638) centre (23, 71.5) ccw
  arc A80 (-17.170094, 149.796638) -> (-17.546037, 147.401376) centre (-16.485377, 148.462036) ccw
  line L46 (-17.546037, 147.401376) -> (-11.559255, 141.414594)
  arc A81 (-11.559255, 137.171953) -> (-11.559255, 141.414594) centre (-13.680575, 139.293273) ccw
  line L47 (-11.559255, 137.171953) -> (-13.574509, 135.156699)
  circle A82 centre (-41.936507, 55) radius 1
  arc A83 (-44.936507, 55) -> (-41.111237, 52.115745) centre (-41.936507, 55) ccw
  circle A84 centre (6.5, 6.563493) radius 1
  line L48 (-44.936507, 55) -> (-44.936507, 57.853553)
  line L49 (-45.936507, 58.853553) -> (-46, 58.853553)
  line L50 (-47, 57.853553) -> (-47, 46)
  line L51 (-25.062149, 24.852065) -> (-38.148194, 11.76602)
  arc A85 (-39.883368, 51.457993) -> (-25.041356, 26.244856) centre (23, 71.5) ccw
  line L52 (-48, 45) -> (-51.631295, 45)
  arc A86 (-54.47978, 33.040492) -> (-39.578754, 11.782754) centre (23, 71.5) ccw
  circle A87 centre (-56.548727, 43) radius 4 construction
  arc A88 (-53.793418, 34.46295) -> (-51.16789, 38.871248) centre (-54.526174, 37.885386) ccw
  line L53 (-52.590805, 43.718325) -> (-51.16789, 38.871248)
  arc A89 (-60.76863, 44.540462) -> (-3.959538, -12.26863) centre (23, 71.5) ccw
  line L54 (-39.225397, 9.274603) -> (-22.608387, 25.891613) construction
  arc A90 (-46, 58.853553) -> (-47, 57.853553) centre (-46, 57.853553) ccw
  arc A91 (-44.936507, 57.853553) -> (-45.936507, 58.853553) centre (-45.936507, 57.853553) ccw
  arc A92 (-39.883368, 51.457993) -> (-41.111237, 52.115745) centre (-40.836146, 51.154326) ccw
  arc A93 (-48, 45) -> (-47, 46) centre (-48, 46) ccw
  arc A94 (-51.631295, 45) -> (-52.590805, 43.718325) centre (-51.631295, 44) ccw
  arc A95 (-53.793418, 34.46295) -> (-54.47978, 33.040492) centre (-53.58406, 33.485111) ccw
  arc A96 (-25.062149, 24.852065) -> (-25.041356, 26.244856) centre (-25.769256, 25.559172) ccw
  arc A97 (-39.578754, 11.782754) -> (-38.148194, 11.76602) centre (-38.855301, 12.473127) ccw
  arc A98 (3.615745, 7.388763) -> (6.5, 3.563493) centre (6.5, 6.563493) ccw
  line L55 (6.5, 3.563493) -> (9.353553, 3.563493)
  line L56 (10.353553, 2.563493) -> (10.353553, 2.5)
  line L57 (9.353553, 1.5) -> (-2.5, 1.5)
  line L58 (-23.647935, 23.437851) -> (-36.73398, 10.351806)
  arc A99 (-22.255144, 23.458644) -> (2.957993, 8.616632) centre (23, 71.5) ccw
  line L59 (-3.5, 0.5) -> (-3.5, -3.131295)
  arc A100 (-36.717246, 8.921246) -> (-15.459508, -5.97978) centre (23, 71.5) ccw
  arc A101 (-9.628752, -2.66789) -> (-14.03705, -5.293418) centre (-10.614614, -6.026174) ccw
  line L60 (-4.781675, -4.090805) -> (-9.628752, -2.66789)
  arc A102 (9.353553, 1.5) -> (10.353553, 2.5) centre (9.353553, 2.5) ccw
  arc A103 (10.353553, 2.563493) -> (9.353553, 3.563493) centre (9.353553, 2.563493) ccw
  arc A104 (3.615745, 7.388763) -> (2.957993, 8.616632) centre (2.654326, 7.663854) ccw
  arc A105 (-2.5, 1.5) -> (-3.5, 0.5) centre (-2.5, 0.5) ccw
  arc A106 (-4.781675, -4.090805) -> (-3.5, -3.131295) centre (-4.5, -3.131295) ccw
  arc A107 (-15.459508, -5.97978) -> (-14.03705, -5.293418) centre (-15.014889, -5.08406) ccw
  arc A108 (-22.255144, 23.458644) -> (-23.647935, 23.437851) centre (-22.940828, 22.730744) ccw
  arc A109 (-36.73398, 10.351806) -> (-36.717246, 8.921246) centre (-36.026873, 9.644699) ccw
  arc A110 (-57.032735, 104.317851) -> (-58.903641, 99.321637) centre (23, 71.5) ccw
  line L61 (-57.956779, 98) -> (-51.169048, 98)
  line L62 (-59.340755, 96.5) -> (-50.5, 96.5)
  line L63 (-55.400394, 104.64556) -> (-50.461941, 99.707107)
  line L64 (-49.182361, 100.548847) -> (-53.839215, 105.205701)
  arc A111 (-55.400394, 104.64556) -> (-57.032735, 104.317851) centre (-56.107501, 103.938454) ccw
  arc A112 (-58.903641, 99.321637) -> (-57.956779, 98) centre (-57.956779, 99) ccw
  arc A113 (-51.169048, 98) -> (-50.461941, 99.707107) centre (-51.169048, 99) ccw
  arc A114 (-36.24577, 100.585027) -> (-40.073462, 90.935494) centre (23, 71.5) ccw
  line L65 (-36.436326, 101.732816) -> (-39.949592, 105.246082)
  arc A115 (-40.987544, 90.230835) -> (-44.725419, 85.364016) centre (-40.821239, 86.234294) ccw
  line L66 (-45.701463, 84.146447) -> (-46, 84.146447)
  line L67 (-47, 85.146447) -> (-47, 99.195674)
  line L68 (-46.707107, 99.902781) -> (-41.363805, 105.246082)
  line L69 (-46.914594, 106.059255) -> (-52.901376, 112.046037)
  line L70 (-40.656699, 108.074509) -> (-42.671953, 106.059255)
  arc A116 (-39.949592, 105.246082) -> (-41.363805, 105.246082) centre (-40.656699, 104.538975) ccw
  arc A117 (-36.24577, 100.585027) -> (-36.436326, 101.732816) centre (-37.143433, 101.025709) ccw
  arc A118 (-46.707107, 99.902781) -> (-47, 99.195674) centre (-46, 99.195674) ccw
  arc A119 (-47, 85.146447) -> (-46, 84.146447) centre (-46, 85.146447) ccw
  arc A120 (-45.701463, 84.146447) -> (-44.725419, 85.364016) centre (-45.701463, 85.146447) ccw
  arc A121 (-40.987544, 90.230835) -> (-40.073462, 90.935494) centre (-41.02912, 91.229971) ccw
  line L71 (-27.115604, 121.615604) -> (73.115604, 21.384396) construction
  line L72 (-39.225397, 9.274603) -> (85.225397, 133.725397) construction
  arc A122 (-4.821637, 153.403641) -> (-9.817851, 151.532735) centre (23, 71.5) ccw
  line L73 (-3.5, 152.456779) -> (-3.5, 145.669048)
  line L74 (-10.14556, 149.900394) -> (-5.207107, 144.961941)
  arc A123 (-9.817851, 151.532735) -> (-10.14556, 149.900394) centre (-9.438454, 150.607501) ccw
  arc A124 (-3.5, 152.456779) -> (-4.821637, 153.403641) centre (-4.5, 152.456779) ccw
  arc A125 (-5.207107, 144.961941) -> (-3.5, 145.669048) centre (-4.5, 145.669048) ccw
  arc A126 (3.564506, 134.573462) -> (-6.085027, 130.74577) centre (23, 71.5) ccw
  line L75 (-7.232816, 130.936326) -> (-10.746082, 134.449592)
  arc A127 (9.135984, 139.225419) -> (4.269165, 135.487544) centre (8.265706, 135.321239) ccw
  line L76 (10.353553, 140.201463) -> (10.353553, 140.5)
  line L77 (9.353553, 141.5) -> (-4.695674, 141.5)
  line L78 (-5.402781, 141.207107) -> (-10.746082, 135.863805)
  arc A128 (-10.746082, 135.863805) -> (-10.746082, 134.449592) centre (-10.038975, 135.156699) ccw
  arc A129 (-7.232816, 130.936326) -> (-6.085027, 130.74577) centre (-6.525709, 131.643433) ccw
  arc A130 (-4.695674, 141.5) -> (-5.402781, 141.207107) centre (-4.695674, 140.5) ccw
  arc A131 (10.353553, 140.5) -> (9.353553, 141.5) centre (9.353553, 140.5) ccw
  arc A132 (9.135984, 139.225419) -> (10.353553, 140.201463) centre (9.353553, 140.201463) ccw
  arc A133 (3.564506, 134.573462) -> (4.269165, 135.487544) centre (3.270029, 135.52912) ccw
  arc A134 (50.821637, -10.403641) -> (55.817851, -8.532735) centre (23, 71.5) ccw
  line L79 (49.5, -9.456779) -> (49.5, -2.669048)
  line L80 (56.14556, -6.900394) -> (51.207107, -1.961941)
  arc A135 (55.817851, -8.532735) -> (56.14556, -6.900394) centre (55.438454, -7.607501) ccw
  arc A136 (49.5, -9.456779) -> (50.821637, -10.403641) centre (50.5, -9.456779) ccw
  arc A137 (51.207107, -1.961941) -> (49.5, -2.669048) centre (50.5, -2.669048) ccw
  arc A138 (42.435494, 8.426538) -> (52.085027, 12.25423) centre (23, 71.5) ccw
  line L81 (53.232816, 12.063674) -> (56.746082, 8.550408)
  arc A139 (36.864016, 3.774581) -> (41.730835, 7.512456) centre (37.734294, 7.678761) ccw
  line L82 (35.646447, 2.798537) -> (35.646447, 2.5)
  line L83 (36.646447, 1.5) -> (50.695674, 1.5)
  line L84 (51.402781, 1.792893) -> (56.746082, 7.136195)
  arc A140 (56.746082, 7.136195) -> (56.746082, 8.550408) centre (56.038975, 7.843301) ccw
  arc A141 (53.232816, 12.063674) -> (52.085027, 12.25423) centre (52.525709, 11.356567) ccw
  arc A142 (50.695674, 1.5) -> (51.402781, 1.792893) centre (50.695674, 2.5) ccw
  arc A143 (35.646447, 2.5) -> (36.646447, 1.5) centre (36.646447, 2.5) ccw
  arc A144 (36.864016, 3.774581) -> (35.646447, 2.798537) centre (36.646447, 2.798537) ccw
  arc A145 (42.435494, 8.426538) -> (41.730835, 7.512456) centre (42.729971, 7.47088) ccw
  arc A146 (101.400394, 38.35444) -> (103.032735, 38.682149) centre (102.107501, 39.061546) ccw
  arc A147 (103.032735, 38.682149) -> (104.903641, 43.678363) centre (23, 71.5) ccw
  arc A148 (104.903641, 43.678363) -> (103.956779, 45) centre (103.956779, 44) ccw
  line L85 (103.956779, 45) -> (97.169048, 45)
  arc A149 (97.169048, 45) -> (96.461941, 43.292893) centre (97.169048, 44) ccw
  line L86 (101.400394, 38.35444) -> (96.461941, 43.292893)
  arc A150 (85.949592, 37.753918) -> (87.363805, 37.753918) centre (86.656699, 38.461025) ccw
  line L87 (92.707107, 43.097219) -> (87.363805, 37.753918)
  arc A151 (92.707107, 43.097219) -> (93, 43.804326) centre (92, 43.804326) ccw
  line L88 (93, 57.853553) -> (93, 43.804326)
  arc A152 (93, 57.853553) -> (92, 58.853553) centre (92, 57.853553) ccw
  line L89 (91.701463, 58.853553) -> (92, 58.853553)
  arc A153 (91.701463, 58.853553) -> (90.725419, 57.635984) centre (91.701463, 57.853553) ccw
  arc A154 (86.987544, 52.769165) -> (86.073462, 52.064506) centre (87.02912, 51.770029) ccw
  arc A155 (86.987544, 52.769165) -> (90.725419, 57.635984) centre (86.821239, 56.765706) ccw
  arc A156 (82.24577, 42.414973) -> (86.073462, 52.064506) centre (23, 71.5) ccw
  line L90 (82.436326, 41.267184) -> (85.949592, 37.753918)
  arc A157 (82.24577, 42.414973) -> (82.436326, 41.267184) centre (83.143433, 41.974291) ccw
  arc A158 (42.384255, 135.611237) -> (39.5, 139.436507) centre (39.5, 136.436507) ccw
  line L91 (39.5, 139.436507) -> (36.646447, 139.436507)
  line L92 (35.646447, 140.436507) -> (35.646447, 140.5)
  line L93 (36.646447, 141.5) -> (48.5, 141.5)
  line L94 (69.647935, 119.562149) -> (82.73398, 132.648194)
  arc A159 (68.255144, 119.541356) -> (43.042007, 134.383368) centre (23, 71.5) ccw
  line L95 (49.5, 142.5) -> (49.5, 146.131295)
  arc A160 (82.717246, 134.078754) -> (61.459508, 148.97978) centre (23, 71.5) ccw
  arc A161 (55.628752, 145.66789) -> (60.03705, 148.293418) centre (56.614614, 149.026174) ccw
  line L96 (50.781675, 147.090805) -> (55.628752, 145.66789)
  arc A162 (36.646447, 141.5) -> (35.646447, 140.5) centre (36.646447, 140.5) ccw
  arc A163 (35.646447, 140.436507) -> (36.646447, 139.436507) centre (36.646447, 140.436507) ccw
  arc A164 (42.384255, 135.611237) -> (43.042007, 134.383368) centre (43.345674, 135.336146) ccw
  arc A165 (48.5, 141.5) -> (49.5, 142.5) centre (48.5, 142.5) ccw
  arc A166 (50.781675, 147.090805) -> (49.5, 146.131295) centre (50.5, 146.131295) ccw
  arc A167 (61.459508, 148.97978) -> (60.03705, 148.293418) centre (61.014889, 148.08406) ccw
  arc A168 (68.255144, 119.541356) -> (69.647935, 119.562149) centre (68.940828, 120.269256) ccw
  arc A169 (82.73398, 132.648194) -> (82.717246, 134.078754) centre (82.026873, 133.355301) ccw
  line L97 (91.936507, 84.146447) -> (92, 84.146447)
  arc A170 (92, 84.146447) -> (93, 85.146447) centre (92, 85.146447) ccw
  arc A171 (90.936507, 85.146447) -> (91.936507, 84.146447) centre (91.936507, 85.146447) ccw
  line L98 (90.936507, 88) -> (90.936507, 85.146447)
  arc A172 (90.936507, 88) -> (87.111237, 90.884255) centre (87.936507, 88) ccw
  line L99 (93, 85.146447) -> (93, 97)
  line L100 (94, 98) -> (97.631295, 98)
  arc A173 (94, 98) -> (93, 97) centre (94, 97) ccw
  arc A174 (97.631295, 98) -> (98.590805, 99.281675) centre (97.631295, 99) ccw
  line L101 (98.590805, 99.281675) -> (97.16789, 104.128752)
  arc A175 (99.793418, 108.53705) -> (97.16789, 104.128752) centre (100.526174, 105.114614) ccw
  arc A176 (99.793418, 108.53705) -> (100.47978, 109.959508) centre (99.58406, 109.514889) ccw
  arc A177 (100.47978, 109.959508) -> (85.578754, 131.217246) centre (23, 71.5) ccw
  arc A178 (85.578754, 131.217246) -> (84.148194, 131.23398) centre (84.855301, 130.526873) ccw
  line L102 (71.062149, 118.147935) -> (84.148194, 131.23398)
  arc A179 (71.062149, 118.147935) -> (71.041356, 116.755144) centre (71.769256, 117.440828) ccw
  arc A180 (85.883368, 91.542007) -> (71.041356, 116.755144) centre (23, 71.5) ccw
  arc A181 (85.883368, 91.542007) -> (87.111237, 90.884255) centre (86.836146, 91.845674) ccw
  arc A182 (-60.76863, 98.459538) -> (-59.340755, 96.5) centre (-59.340755, 98) ccw
  line L103 (-59.340755, 96.5) -> (-50.5, 96.5)
  arc A183 (-48.5, 94.5) -> (-50.5, 96.5) centre (-50.5, 94.5) ccw
  arc A184 (-2, 145) -> (0, 143) centre (0, 145) ccw
  line L104 (-2, 145) -> (-2, 153.840755)
  arc A185 (-2, 153.840755) -> (-3.959538, 155.26863) centre (-3.5, 153.840755) ccw
  point P0 (23, 5.5)
  point P1 (-24.370797, 25.543416)
  point P2 (-38.867756, 11.046458)
  point P3 (-24.370797, 25.543416)
  point P4 (-38.867756, 11.046458)
  point P5 (-56.452807, 105.697973)
  point P6 (-59.340755, 98)
  point P7 (-59.340755, 98)
  point P8 (-35.927693, 101.224183)
  point P9 (-44.233115, 84.146447)
  dimension "d71" = 1.5
  dimension "d72" = 3
  dimension "d73" = 1.5
  dimension "d74" = 1.5
  dimension "d75" = 1.5
  dimension "d76" = 8
  dimension "d77" = 1.5
  dimension "d79" = 1.5
  dimension "d80" = 1
  dimension "d81" = 1
  dimension "d91" = 1.5
  dimension "d93" = 1.5
  dimension "d94" = 1
  dimension "d95" = 1.5
  dimension "d96" = 1.5
  dimension "d97" = 1.5
  dimension "d98" = 1.5
  dimension "d99" = 1.5
  dimension "d100" = 1.5
  dimension "d101" = 1
  constraints: 211 point on circle, 171 symmetric about line, 102 end point, 97 centre point, 37 tangent, 14 equal radius, 13 point on line, 10 coincident, 5 parallel, 3 horizontal, 3 perpendicular, 2 midpoint, 1 concentric, 1 vertical, 72 other
  measures "d71" radial gap between concentric circles of A7 A85
  measures "d72" radius of A83
  measures "d73" distance edge to line of A27 L49
  measures "d74" distance between parallel lines of L25 L50
  measures "d75" distance between parallel lines of L26 L52
  measures "d76" diameter of A87
  measures "d77" radial gap between concentric circles of A53 A86
  measures "d79" radial gap between concentric circles of A88 A38
  measures "d80" distance between parallel lines of L54 L51
  measures "d81" radius of A90
  measures "d91" radial gap between concentric circles of A50 A110
  measures "d93" distance between parallel lines of L64 L63
  measures "d94" radius of A111
  measures "d95" radial gap between concentric circles of A114 A11
  measures "d96" radial gap between concentric circles of A115 A9
  measures "d97" distance edge to line of A46 L65